Autodesk Fusion 360 part; units mm, degrees
(part 2 of 3)
pattern_linear "Serie R1" count 32 spacing 6 along (-1, 0, 0) count 32 spacing 6 along (0, 1, 0) of bodies 2 makes body 3 at (85.6178, -93.5827, 13.8667) makes body 4 at (79.6178, -93.5827, 13.8667) makes body 5 at (73.6178, -93.5827, 13.8667) makes body 6 at (67.6178, -93.5827, 13.8667) makes body 7 at (61.6178, -93.5827, 13.8667) makes body 8 at (55.6178, -93.5827, 13.8667) makes body 9 at (49.6178, -93.5827, 13.8667) makes body 10 at (43.6178, -93.5827, 13.8667) makes body 11 at (37.6178, -93.5827, 13.8667) makes body 12 at (31.6178, -93.5827, 13.8667) makes body 13 at (25.6178, -93.5827, 13.8667) makes body 14 at (19.6178, -93.5827, 13.8667) makes body 15 at (13.6178, -93.5827, 13.8667) makes body 16 at (10.4095, -93.513, 13.8667) makes body 17 at (4.4095, -93.513, 13.8667) makes body 18 at (-1.5905, -93.513, 13.8667) makes body 19 at (-10.3822, -93.5827, 13.8667) makes body 20 at (-16.3822, -93.5827, 13.8667) makes body 21 at (-22.3822, -93.5827, 13.8667) makes body 22 at (-28.3822, -93.5827, 13.8667) makes body 23 at (-34.3822, -93.5827, 13.8667) makes body 24 at (-40.3822, -93.5827, 13.8667) makes body 25 at (-46.3822, -93.5827, 13.8667) makes body 26 at (-52.3822, -93.5827, 13.8667) makes body 27 at (-58.3822, -93.5827, 13.8667) makes body 28 at (-64.3822, -93.5827, 13.8667) makes body 29 at (-70.3822, -93.5827, 13.8667) makes body 30 at (-76.3822, -93.5827, 13.8667) makes body 31 at (-82.3822, -93.5827, 13.8667) makes body 32 at (-88.3822, -93.5827, 13.8667) makes body 33 at (-94.3822, -93.5827, 13.8667) makes body 34 at (91.6178, -87.5827, 13.8667) makes body 35 at (85.6178, -87.5827, 13.8667) makes body 36 at (79.6178, -87.5827, 13.8667) makes body 37 at (73.6178, -87.5827, 13.8667) makes body 38 at (67.6178, -87.5827, 13.8667) makes body 39 at (61.6178, -87.5827, 13.8667) makes body 40 at (55.6178, -87.5827, 13.8667) makes body 41 at (49.6178, -87.5827, 13.8667) makes body 42 at (43.6178, -87.5827, 13.8667) makes body 43 at (37.6178, -87.5827, 13.8667) makes body 44 at (31.6178, -87.5827, 13.8667) makes body 45 at (25.6178, -87.5827, 13.8667) makes body 46 at (19.6178, -87.5827, 13.8667) makes body 47 at (13.6178, -87.5827, 13.8667) makes body 48 at (10.4095, -87.513, 13.8667) makes body 49 at (4.4095, -87.513, 13.8667) makes body 50 at (-1.5905, -87.513, 13.8667) makes body 51 at (-10.3822, -87.5827, 13.8667) makes body 52 at (-16.3822, -87.5827, 13.8667) makes body 53 at (-22.3822, -87.5827, 13.8667) makes body 54 at (-28.3822, -87.5827, 13.8667) makes body 55 at (-34.3822, -87.5827, 13.8667) makes body 56 at (-40.3822, -87.5827, 13.8667) makes body 57 at (-46.3822, -87.5827, 13.8667) makes body 58 at (-52.3822, -87.5827, 13.8667) makes body 59 at (-58.3822, -87.5827, 13.8667) makes body 60 at (-64.3822, -87.5827, 13.8667) makes body 61 at (-70.3822, -87.5827, 13.8667) makes body 62 at (-76.3822, -87.5827, 13.8667) makes body 63 at (-82.3822, -87.5827, 13.8667) makes body 64 at (-88.3822, -87.5827, 13.8667) makes body 65 at (-94.3822, -87.5827, 13.8667) makes body 66 at (91.6178, -81.5827, 13.8667) makes body 67 at (85.6178, -81.5827, 13.8667) makes body 68 at (79.6178, -81.5827, 13.8667) makes body 69 at (73.6178, -81.5827, 13.8667) makes body 70 at (67.6178, -81.5827, 13.8667) makes body 71 at (61.6178, -81.5827, 13.8667) makes body 72 at (55.6178, -81.5827, 13.8667) makes body 73 at (49.6178, -81.5827, 13.8667) makes body 74 at (43.6178, -81.5827, 13.8667) makes body 75 at (37.6178, -81.5827, 13.8667) makes body 76 at (31.6178, -81.5827, 13.8667) makes body 77 at (25.6178, -81.5827, 13.8667) makes body 78 at (19.6178, -81.5827, 13.8667) makes body 79 at (13.6178, -81.5827, 13.8667) makes body 80 at (10.4095, -81.513, 13.8667) makes body 81 at (4.4095, -81.513, 13.8667) makes body 82 at (-1.5905, -81.513, 13.8667) makes body 83 at (-10.3822, -81.5827, 13.8667) makes body 84 at (-16.3822, -81.5827, 13.8667) makes body 85 at (-22.3822, -81.5827, 13.8667) makes body 86 at (-28.3822, -81.5827, 13.8667) makes body 87 at (-34.3822, -81.5827, 13.8667) makes body 88 at (-40.3822, -81.5827, 13.8667) makes body 89 at (-46.3822, -81.5827, 13.8667) makes body 90 at (-52.3822, -81.5827, 13.8667) makes body 91 at (-58.3822, -81.5827, 13.8667) makes body 92 at (-64.3822, -81.5827, 13.8667) makes body 93 at (-70.3822, -81.5827, 13.8667) makes body 94 at (-76.3822, -81.5827, 13.8667) makes body 95 at (-82.3822, -81.5827, 13.8667) makes body 96 at (-88.3822, -81.5827, 13.8667) makes body 97 at (-94.3822, -81.5827, 13.8667) makes body 98 at (91.6178, -75.5827, 13.8667) makes body 99 at (85.6178, -75.5827, 13.8667) makes body 100 at (79.6178, -75.5827, 13.8667) makes body 101 at (73.6178, -75.5827, 13.8667) makes body 102 at (67.6178, -75.5827, 13.8667) makes body 103 at (61.6178, -75.5827, 13.8667) makes body 104 at (55.6178, -75.5827, 13.8667) makes body 105 at (49.6178, -75.5827, 13.8667) makes body 106 at (43.6178, -75.5827, 13.8667) makes body 107 at (37.6178, -75.5827, 13.8667) makes body 108 at (31.6178, -75.5827, 13.8667) makes body 109 at (25.6178, -75.5827, 13.8667) makes body 110 at (19.6178, -75.5827, 13.8667) makes body 111 at (13.6178, -75.5827, 13.8667) makes body 112 at (10.4095, -75.513, 13.8667) makes body 113 at (4.4095, -75.513, 13.8667) makes body 114 at (-1.5905, -75.513, 13.8667) makes body 115 at (-10.3822, -75.5827, 13.8667) makes body 116 at (-16.3822, -75.5827, 13.8667) makes body 117 at (-22.3822, -75.5827, 13.8667) makes body 118 at (-28.3822, -75.5827, 13.8667) makes body 119 at (-34.3822, -75.5827, 13.8667) makes body 120 at (-40.3822, -75.5827, 13.8667) makes body 121 at (-46.3822, -75.5827, 13.8667) makes body 122 at (-52.3822, -75.5827, 13.8667) makes body 123 at (-58.3822, -75.5827, 13.8667) makes body 124 at (-64.3822, -75.5827, 13.8667) makes body 125 at (-70.3822, -75.5827, 13.8667) makes body 126 at (-76.3822, -75.5827, 13.8667) makes body 127 at (-82.3822, -75.5827, 13.8667) makes body 128 at (-88.3822, -75.5827, 13.8667) makes body 129 at (-94.3822, -75.5827, 13.8667) makes body 130 at (91.6178, -69.5827, 13.8667) makes body 131 at (85.6178, -69.5827, 13.8667) makes body 132 at (79.6178, -69.5827, 13.8667) makes body 133 at (73.6178, -69.5827, 13.8667) makes body 134 at (67.6178, -69.5827, 13.8667) makes body 135 at (61.6178, -69.5827, 13.8667) makes body 136 at (55.6178, -69.5827, 13.8667) makes body 137 at (49.6178, -69.5827, 13.8667) makes body 138 at (43.6178, -69.5827, 13.8667) makes body 139 at (37.6178, -69.5827, 13.8667) makes body 140 at (31.6178, -69.5827, 13.8667) makes body 141 at (25.6178, -69.5827, 13.8667) makes body 142 at (19.6178, -69.5827, 13.8667) makes body 143 at (13.6178, -69.5827, 13.8667) makes body 144 at (10.4095, -69.513, 13.8667) makes body 145 at (4.4095, -69.513, 13.8667) makes body 146 at (-1.5905, -69.513, 13.8667) makes body 147 at (-10.3822, -69.5827, 13.8667) makes body 148 at (-16.3822, -69.5827, 13.8667) makes body 149 at (-22.3822, -69.5827, 13.8667) makes body 150 at (-28.3822, -69.5827, 13.8667) makes body 151 at (-34.3822, -69.5827, 13.8667) makes body 152 at (-40.3822, -69.5827, 13.8667) makes body 153 at (-46.3822, -69.5827, 13.8667) makes body 154 at (-52.3822, -69.5827, 13.8667) makes body 155 at (-58.3822, -69.5827, 13.8667) makes body 156 at (-64.3822, -69.5827, 13.8667) makes body 157 at (-70.3822, -69.5827, 13.8667) makes body 158 at (-76.3822, -69.5827, 13.8667) makes body 159 at (-82.3822, -69.5827, 13.8667) makes body 160 at (-88.3822, -69.5827, 13.8667) makes body 161 at (-94.3822, -69.5827, 13.8667) makes body 162 at (94.3822, -62.4173, 13.8667) makes body 163 at (88.3822, -62.4173, 13.8667) makes body 164 at (82.3822, -62.4173, 13.8667) makes body 165 at (76.3822, -62.4173, 13.8667) makes body 166 at (70.3822, -62.4173, 13.8667) makes body 167 at (64.3822, -62.4173, 13.8667) makes body 168 at (58.3822, -62.4173, 13.8667) makes body 169 at (52.3822, -62.4173, 13.8667) makes body 170 at (46.3822, -62.4173, 13.8667) makes body 171 at (40.3822, -62.4173, 13.8667) makes body 172 at (34.3822, -62.4173, 13.8667) makes body 173 at (28.3822, -62.4173, 13.8667) makes body 174 at (22.3822, -62.4173, 13.8667) makes body 175 at (16.3822, -62.4173, 13.8667) makes body 176 at (10.3822, -62.4173, 13.8667) makes body 177 at (4.3822, -62.4173, 13.8667) makes body 178 at (-1.6178, -62.4173, 13.8667) makes body 179 at (-7.6178, -62.4173, 13.8667) makes body 180 at (-13.6178, -62.4173, 13.8667) makes body 181 at (-19.6178, -62.4173, 13.8667) makes body 182 at (-25.6178, -62.4173, 13.8667) makes body 183 at (-31.6178, -62.4173, 13.8667) makes body 184 at (-37.6178, -62.4173, 13.8667) makes body 185 at (-43.6178, -62.4173, 13.8667) makes body 186 at (-49.6178, -62.4173, 13.8667) makes body 187 at (-55.6178, -62.4173, 13.8667) makes body 188 at (-61.6178, -62.4173, 13.8667) makes body 189 at (-67.6178, -62.4173, 13.8667) makes body 190 at (-73.6178, -62.4173, 13.8667) makes body 191 at (-79.6178, -62.4173, 13.8667) makes body 192 at (-85.6178, -62.4173, 13.8667) makes body 193 at (-91.6178, -62.4173, 13.8667) makes body 194 at (94.3822, -56.4173, 13.8667) makes body 195 at (88.3822, -56.4173, 13.8667) makes body 196 at (82.3822, -56.4173, 13.8667) makes body 197 at (76.3822, -56.4173, 13.8667) makes body 198 at (70.3822, -56.4173, 13.8667) makes body 199 at (64.3822, -56.4173, 13.8667) makes body 200 at (58.3822, -56.4173, 13.8667) makes body 201 at (52.3822, -56.4173, 13.8667) makes body 202 at (46.3822, -56.4173, 13.8667) makes body 203 at (40.3822, -56.4173, 13.8667) makes body 204 at (34.3822, -56.4173, 13.8667) makes body 205 at (28.3822, -56.4173, 13.8667) makes body 206 at (22.3822, -56.4173, 13.8667) makes body 207 at (16.3822, -56.4173, 13.8667) makes body 208 at (10.3822, -56.4173, 13.8667) makes body 209 at (4.3822, -56.4173, 13.8667) makes body 210 at (-1.6178, -56.4173, 13.8667) makes body 211 at (-7.6178, -56.4173, 13.8667) makes body 212 at (-13.6178, -56.4173, 13.8667) makes body 213 at (-19.6178, -56.4173, 13.8667) makes body 214 at (-25.6178, -56.4173, 13.8667) makes body 215 at (-31.6178, -56.4173, 13.8667) makes body 216 at (-37.6178, -56.4173, 13.8667) makes body 217 at (-43.6178, -56.4173, 13.8667) makes body 218 at (-49.6178, -56.4173, 13.8667) makes body 219 at (-55.6178, -56.4173, 13.8667) makes body 220 at (-61.6178, -56.4173, 13.8667) makes body 221 at (-67.6178, -56.4173, 13.8667) makes body 222 at (-73.6178, -56.4173, 13.8667) makes body 223 at (-79.6178, -56.4173, 13.8667) makes body 224 at (-85.6178, -56.4173, 13.8667) makes body 225 at (-91.6178, -56.4173, 13.8667) makes body 226 at (94.3822, -50.4173, 13.8667) makes body 227 at (88.3822, -50.4173, 13.8667) makes body 228 at (82.3822, -50.4173, 13.8667) makes body 229 at (76.3822, -50.4173, 13.8667) makes body 230 at (70.3822, -50.4173, 13.8667) makes body 231 at (64.3822, -50.4173, 13.8667) makes body 232 at (58.3822, -50.4173, 13.8667) makes body 233 at (52.3822, -50.4173, 13.8667) makes body 234 at (46.3822, -50.4173, 13.8667) makes body 235 at (40.3822, -50.4173, 13.8667) makes body 236 at (34.3822, -50.4173, 13.8667) makes body 237 at (28.3822, -50.4173, 13.8667) makes body 238 at (22.3822, -50.4173, 13.8667) makes body 239 at (16.3822, -50.4173, 13.8667) makes body 240 at (10.3822, -50.4173, 13.8667) makes body 241 at (4.3822, -50.4173, 13.8667) makes body 242 at (-1.6178, -50.4173, 13.8667) makes body 243 at (-7.6178, -50.4173, 13.8667) makes body 244 at (-13.6178, -50.4173, 13.8667) makes body 245 at (-19.6178, -50.4173, 13.8667) makes body 246 at (-25.6178, -50.4173, 13.8667) makes body 247 at (-31.6178, -50.4173, 13.8667) makes body 248 at (-37.6178, -50.4173, 13.8667) makes body 249 at (-43.6178, -50.4173, 13.8667) makes body 250 at (-49.6178, -50.4173, 13.8667) makes body 251 at (-55.6178, -50.4173, 13.8667) makes body 252 at (-61.6178, -50.4173, 13.8667) makes body 253 at (-67.6178, -50.4173, 13.8667) makes body 254 at (-73.6178, -50.4173, 13.8667) makes body 255 at (-79.6178, -50.4173, 13.8667) makes body 256 at (-85.6178, -50.4173, 13.8667) makes body 257 at (-91.6178, -50.4173, 13.8667) makes body 258 at (94.3822, -44.4173, 13.8667) makes body 259 at (88.3822, -44.4173, 13.8667) makes body 260 at (82.3822, -44.4173, 13.8667) makes body 261 at (76.3822, -44.4173, 13.8667) makes body 262 at (70.3822, -44.4173, 13.8667) makes body 263 at (64.3822, -44.4173, 13.8667) makes body 264 at (58.3822, -44.4173, 13.8667) makes body 265 at (52.3822, -44.4173, 13.8667) makes body 266 at (46.3822, -44.4173, 13.8667) makes body 267 at (40.3822, -44.4173, 13.8667) makes body 268 at (34.3822, -44.4173, 13.8667) makes body 269 at (28.3822, -44.4173, 13.8667) makes body 270 at (22.3822, -44.4173, 13.8667) makes body 271 at (16.3822, -44.4173, 13.8667) makes body 272 at (10.3822, -44.4173, 13.8667) makes body 273 at (4.3822, -44.4173, 13.8667) makes body 274 at (-1.6178, -44.4173, 13.8667) makes body 275 at (-7.6178, -44.4173, 13.8667) makes body 276 at (-13.6178, -44.4173, 13.8667) makes body 277 at (-19.6178, -44.4173, 13.8667) makes body 278 at (-25.6178, -44.4173, 13.8667) makes body 279 at (-31.6178, -44.4173, 13.8667) makes body 280 at (-37.6178, -44.4173, 13.8667) makes body 281 at (-43.6178, -44.4173, 13.8667) makes body 282 at (-49.6178, -44.4173, 13.8667) makes body 283 at (-55.6178, -44.4173, 13.8667) makes body 284 at (-61.6178, -44.4173, 13.8667) makes body 285 at (-67.6178, -44.4173, 13.8667) makes body 286 at (-73.6178, -44.4173, 13.8667) makes body 287 at (-79.6178, -44.4173, 13.8667) makes body 288 at (-85.6178, -44.4173, 13.8667) makes body 289 at (-91.6178, -44.4173, 13.8667) makes body 290 at (94.3822, -38.4173, 13.8667) makes body 291 at (88.3822, -38.4173, 13.8667) makes body 292 at (82.3822, -38.4173, 13.8667) makes body 293 at (76.3822, -38.4173, 13.8667) makes body 294 at (70.3822, -38.4173, 13.8667) makes body 295 at (64.3822, -38.4173, 13.8667) makes body 296 at (58.3822, -38.4173, 13.8667) makes body 297 at (52.3822, -38.4173, 13.8667) makes body 298 at (46.3822, -38.4173, 13.8667) makes body 299 at (40.3822, -38.4173, 13.8667) makes body 300 at (34.3822, -38.4173, 13.8667) makes body 301 at (28.3822, -38.4173, 13.8667) makes body 302 at (22.3822, -38.4173, 13.8667) makes body 303 at (16.3822, -38.4173, 13.8667) makes body 304 at (10.3822, -38.4173, 13.8667) makes body 305 at (4.3822, -38.4173, 13.8667) makes body 306 at (-1.6178, -38.4173, 13.8667) makes body 307 at (-7.6178, -38.4173, 13.8667) makes body 308 at (-13.6178, -38.4173, 13.8667) makes body 309 at (-19.6178, -38.4173, 13.8667) makes body 310 at (-25.6178, -38.4173, 13.8667) makes body 311 at (-31.6178, -38.4173, 13.8667) makes body 312 at (-37.6178, -38.4173, 13.8667) makes body 313 at (-43.6178, -38.4173, 13.8667) makes body 314 at (-49.6178, -38.4173, 13.8667) makes body 315 at (-55.6178, -38.4173, 13.8667) makes body 316 at (-61.6178, -38.4173, 13.8667) makes body 317 at (-67.6178, -38.4173, 13.8667) makes body 318 at (-73.6178, -38.4173, 13.8667) makes body 319 at (-79.6178, -38.4173, 13.8667) makes body 320 at (-85.6178, -38.4173, 13.8667) makes body 321 at (-91.6178, -38.4173, 13.8667) makes body 322 at (94.3822, -32.4173, 13.8667) makes body 323 at (88.3822, -32.4173, 13.8667) makes body 324 at (82.3822, -32.4173, 13.8667) makes body 325 at (76.3822, -32.4173, 13.8667) makes body 326 at (70.3822, -32.4173, 13.8667) makes body 327 at (64.3822, -32.4173, 13.8667) makes body 328 at (58.3822, -32.4173, 13.8667) makes body 329 at (52.3822, -32.4173, 13.8667) makes body 330 at (46.3822, -32.4173, 13.8667) makes body 331 at (40.3822, -32.4173, 13.8667) makes body 332 at (34.3822, -32.4173, 13.8667) makes body 333 at (28.3822, -32.4173, 13.8667) makes body 334 at (22.3822, -32.4173, 13.8667) makes body 335 at (16.3822, -32.4173, 13.8667) makes body 336 at (10.3822, -32.4173, 13.8667) makes body 337 at (4.3822, -32.4173, 13.8667) makes body 338 at (-1.6178, -32.4173, 13.8667) makes body 339 at (-7.6178, -32.4173, 13.8667) makes body 340 at (-13.6178, -32.4173, 13.8667) makes body 341 at (-19.6178, -32.4173, 13.8667) makes body 342 at (-25.6178, -32.4173, 13.8667) makes body 343 at (-31.6178, -32.4173, 13.8667) makes body 344 at (-37.6178, -32.4173, 13.8667) makes body 345 at (-43.6178, -32.4173, 13.8667) makes body 346 at (-49.6178, -32.4173, 13.8667) makes body 347 at (-55.6178, -32.4173, 13.8667) makes body 348 at (-61.6178, -32.4173, 13.8667) makes body 349 at (-67.6178, -32.4173, 13.8667) makes body 350 at (-73.6178, -32.4173, 13.8667) makes body 351 at (-79.6178, -32.4173, 13.8667) makes body 352 at (-85.6178, -32.4173, 13.8667) makes body 353 at (-91.6178, -32.4173, 13.8667) makes body 354 at (92.0075, -28.1247, 13.8667) makes body 355 at (86.0075, -28.1247, 13.8667) makes body 356 at (80.0075, -28.1247, 13.8667) makes body 357 at (74.0075, -28.1247, 13.8667) makes body 358 at (68.0075, -28.1247, 13.8667) makes body 359 at (62.5937, -28.4439, 13.8667) makes body 360 at (56.5937, -28.4439, 13.8667) makes body 361 at (50.5937, -28.4439, 13.8667) makes body 362 at (44.5937, -28.4439, 13.8667) makes body 363 at (38.5937, -28.4439, 13.8667) makes body 364 at (32.5937, -28.4439, 13.8667) makes body 365 at (28.4925, -26.8506, 13.8667) makes body 366 at (22.4925, -26.8506, 13.8667) makes body 367 at (16.4925, -26.8506, 13.8667) makes body 368 at (10.4925, -26.8506, 13.8667) makes body 369 at (1.5075, -26.8506, 13.5333) makes body 370 at (-4.4925, -26.8506, 13.5333) makes body 371 at (-10.4925, -26.8506, 13.5333) makes body 372 at (-13.5075, -26.8506, 13.8667) makes body 373 at (-19.5075, -26.8506, 13.8667) makes body 374 at (-25.5075, -26.8506, 13.8667) makes body 375 at (-33.4063, -28.4439, 13.8667) makes body 376 at (-39.4063, -28.4439, 13.8667) makes body 377 at (-45.4063, -28.4439, 13.8667) makes body 378 at (-51.4063, -28.4439, 13.8667) makes body 379 at (-57.4063, -28.4439, 13.8667) makes body 380 at (-63.4063, -28.4439, 13.8667) makes body 381 at (-69.9925, -28.1247, 13.8667) makes body 382 at (-75.9925, -28.1247, 13.8667) makes body 383 at (-81.9925, -28.1247, 13.8667) makes body 384 at (-87.9925, -28.1247, 13.8667) makes body 385 at (-93.9925, -28.1247, 13.8667) makes body 386 at (92.0075, -22.1247, 13.8667) makes body 387 at (86.0075, -22.1247, 13.8667) makes body 388 at (80.0075, -22.1247, 13.8667) makes body 389 at (74.0075, -22.1247, 13.8667) makes body 390 at (68.0075, -22.1247, 13.8667) makes body 391 at (62.5937, -22.4439, 13.8667) makes body 392 at (56.5937, -22.4439, 13.8667) makes body 393 at (50.5937, -22.4439, 13.8667) makes body 394 at (44.5937, -22.4439, 13.8667) makes body 395 at (38.5937, -22.4439, 13.8667) makes body 396 at (32.5937, -22.4439, 13.8667) makes body 397 at (28.4925, -20.8506, 13.8667) makes body 398 at (22.4925, -20.8506, 13.8667) makes body 399 at (16.4925, -20.8506, 13.8667) makes body 400 at (10.4925, -20.8506, 13.8667) makes body 401 at (1.5075, -20.8506, 13.5333) makes body 402 at (-4.4925, -20.8506, 13.5333) makes body 403 at (-10.4925, -20.8506, 13.5333) makes body 404 at (-13.5075, -20.8506, 13.8667) makes body 405 at (-19.5075, -20.8506, 13.8667) makes body 406 at (-25.5075, -20.8506, 13.8667) makes body 407 at (-33.4063, -22.4439, 13.8667) makes body 408 at (-39.4063, -22.4439, 13.8667) makes body 409 at (-45.4063, -22.4439, 13.8667) makes body 410 at (-51.4063, -22.4439, 13.8667) makes body 411 at (-57.4063, -22.4439, 13.8667) makes body 412 at (-63.4063, -22.4439, 13.8667) makes body 413 at (-69.9925, -22.1247, 13.8667) makes body 414 at (-75.9925, -22.1247, 13.8667) makes body 415 at (-81.9925, -22.1247, 13.8667) makes body 416 at (-87.9925, -22.1247, 13.8667) makes body 417 at (-93.9925, -22.1247, 13.8667) makes body 418 at (92.0075, -16.1247, 13.8667) makes body 419 at (86.0075, -16.1247, 13.8667) makes body 420 at (80.0075, -16.1247, 13.8667) makes body 421 at (74.0075, -16.1247, 13.8667) makes body 422 at (68.0075, -16.1247, 13.8667) makes body 423 at (62.5937, -16.4439, 13.8667) makes body 424 at (56.5937, -16.4439, 13.8667) makes body 425 at (50.5937, -16.4439, 13.8667) makes body 426 at (44.5937, -16.4439, 13.8667) makes body 427 at (38.5937, -16.4439, 13.8667) makes body 428 at (32.5937, -16.4439, 13.8667) makes body 429 at (25.5075, -14.8506, 13.5333) makes body 430 at (19.5075, -14.8506, 13.5333) makes body 431 at (13.5075, -14.8506, 13.5333) makes body 432 at (7.5075, -14.8506, 13.5333) makes body 433 at (1.5075, -14.8506, 13.5333) makes body 434 at (-4.4925, -14.8506, 13.5333) makes body 435 at (-10.4925, -14.8506, 13.5333) makes body 436 at (-16.4925, -14.8506, 13.5333) makes body 437 at (-22.4925, -14.8506, 13.5333) makes body 438 at (-28.4925, -14.8506, 13.5333) makes body 439 at (-33.4063, -16.4439, 13.8667) makes body 440 at (-39.4063, -16.4439, 13.8667) makes body 441 at (-45.4063, -16.4439, 13.8667) makes body 442 at (-51.4063, -16.4439, 13.8667) makes body 443 at (-57.4063, -16.4439, 13.8667) makes body 444 at (-63.4063, -16.4439, 13.8667) makes body 445 at (-69.9925, -16.1247, 13.8667) makes body 446 at (-75.9925, -16.1247, 13.8667) makes body 447 at (-81.9925, -16.1247, 13.8667) makes body 448 at (-87.9925, -16.1247, 13.8667) makes body 449 at (-93.9925, -16.1247, 13.8667) makes body 450 at (92.5937, -10.4439, 13.8667) makes body 451 at (86.5937, -10.4439, 13.8667) makes body 452 at (80.5937, -10.4439, 13.8667) makes body 453 at (74.5937, -10.4439, 13.8667) makes body 454 at (68.5937, -10.4439, 13.8667) makes body 455 at (62.5937, -10.4439, 13.8667) makes body 456 at (56.5937, -10.4439, 13.8667) makes body 457 at (50.5937, -10.4439, 13.8667) makes body 458 at (44.5937, -10.4439, 13.8667) makes body 459 at (38.5937, -10.4439, 13.8667) makes body 460 at (32.5937, -10.4439, 13.8667) makes body 461 at (25.5075, -8.8506, 13.5333) makes body 462 at (19.5075, -8.8506, 13.5333) makes body 463 at (13.5075, -8.8506, 13.5333) makes body 464 at (7.5075, -8.8506, 13.5333) makes body 465 at (1.5075, -8.8506, 13.5333) makes body 466 at (-4.4925, -8.8506, 13.5333) makes body 467 at (-10.4925, -8.8506, 13.5333) makes body 468 at (-16.4925, -8.8506, 13.5333) makes body 469 at (-22.4925, -8.8506, 13.5333) makes body 470 at (-28.4925, -8.8506, 13.5333) makes body 471 at (-33.4063, -10.4439, 13.8667) makes body 472 at (-39.4063, -10.4439, 13.8667) makes body 473 at (-45.4063, -10.4439, 13.8667) makes body 474 at (-51.4063, -10.4439, 13.8667) makes body 475 at (-57.4063, -10.4439, 13.8667) makes body 476 at (-63.4063, -10.4439, 13.8667) makes body 477 at (-69.4063, -10.4439, 13.8667) makes body 478 at (-75.4063, -10.4439, 13.8667) makes body 479 at (-81.4063, -10.4439, 13.8667) makes body 480 at (-87.4063, -10.4439, 13.8667) makes body 481 at (-93.4063, -10.4439, 13.8667) makes body 482 at (91.5075, -2.8506, 13.5333) makes body 483 at (85.5075, -2.8506, 13.5333) makes body 484 at (79.5075, -2.8506, 13.5333) makes body 485 at (73.5075, -2.8506, 13.5333) makes body 486 at (67.5075, -2.8506, 13.5333) makes body 487 at (62.5937, -4.4439, 13.8667) makes body 488 at (56.5937, -4.4439, 13.8667) makes body 489 at (50.5937, -4.4439, 13.8667) makes body 490 at (44.5937, -4.4439, 13.8667) makes body 491 at (38.5937, -4.4439, 13.8667) makes body 492 at (31.5075, -2.8506, 13.5333) makes body 493 at (25.5075, -2.8506, 13.5333) makes body 494 at (19.5075, -2.8506, 13.5333) makes body 495 at (13.5075, -2.8506, 13.5333) makes body 496 at (7.5075, -2.8506, 13.5333) makes body 497 at (1.5075, -2.8506, 13.5333) makes body 498 at (-4.4925, -2.8506, 13.5333) makes body 499 at (-10.4925, -2.8506, 13.5333) makes body 500 at (-16.4925, -2.8506, 13.5333) makes body 501 at (-22.4925, -2.8506, 13.5333) makes body 502 at (-28.4925, -2.8506, 13.5333) makes body 503 at (-33.4063, -4.4439, 13.8667) makes body 504 at (-39.4063, -4.4439, 13.8667) makes body 505 at (-45.4063, -4.4439, 13.8667) makes body 506 at (-51.4063, -4.4439, 13.8667) makes body 507 at (-57.4063, -4.4439, 13.8667) makes body 508 at (-64.4925, -2.8506, 13.5333) makes body 509 at (-70.4925, -2.8506, 13.5333) makes body 510 at (-76.4925, -2.8506, 13.5333) makes body 511 at (-82.4925, -2.8506, 13.5333) makes body 512 at (-88.4925, -2.8506, 13.5333) makes body 513 at (-94.4925, -2.8506, 13.5333) makes body 514 at (91.5075, 3.1494, 13.5333) makes body 515 at (85.5075, 3.1494, 13.5333) makes body 516 at (79.5075, 3.1494, 13.5333) makes body 517 at (73.5075, 3.1494, 13.5333) makes body 518 at (67.5075, 3.1494, 13.5333) makes body 519 at (62.5937, 1.5561, 13.8667) makes body 520 at (56.5937, 1.5561, 13.8667) makes body 521 at (50.5937, 1.5561, 13.8667) makes body 522 at (44.5937, 1.5561, 13.8667) makes body 523 at (38.5937, 1.5561, 13.8667) makes body 524 at (32.5937, 1.5561, 13.8667) makes body 525 at (25.5075, 3.1494, 13.5333) makes body 526 at (19.5075, 3.1494, 13.5333) makes body 527 at (13.5075, 3.1494, 13.5333) makes body 528 at (7.5075, 3.1494, 13.5333) makes body 529 at (1.5075, 3.1494, 13.5333) makes body 530 at (-4.4925, 3.1494, 13.5333) makes body 531 at (-10.4925, 3.1494, 13.5333) makes body 532 at (-16.4925, 3.1494, 13.5333) makes body 533 at (-22.4925, 3.1494, 13.5333) makes body 534 at (-28.4925, 3.1494, 13.5333) makes body 535 at (-33.4063, 1.5561, 13.8667) makes body 536 at (-39.4063, 1.5561, 13.8667) makes body 537 at (-45.4063, 1.5561, 13.8667) makes body 538 at (-51.4063, 1.5561, 13.8667) makes body 539 at (-57.4063, 1.5561, 13.8667) makes body 540 at (-64.4925, 3.1494, 13.5333) makes body 541 at (-70.4925, 3.1494, 13.5333) makes body 542 at (-76.4925, 3.1494, 13.5333) makes body 543 at (-82.4925, 3.1494, 13.5333) makes body 544 at (-88.4925, 3.1494, 13.5333) makes body 545 at (-94.4925, 3.1494, 13.5333) makes body 546 at (92.5937, 7.5561, 13.8667) makes body 547 at (86.5937, 7.5561, 13.8667) makes body 548 at (80.5937, 7.5561, 13.8667) makes body 549 at (74.5937, 7.5561, 13.8667) makes body 550 at (68.5937, 7.5561, 13.8667) makes body 551 at (62.5937, 7.5561, 13.8667) makes body 552 at (56.5937, 7.5561, 13.8667) makes body 553 at (50.5937, 7.5561, 13.8667) makes body 554 at (44.5937, 7.5561, 13.8667) makes body 555 at (38.5937, 7.5561, 13.8667) makes body 556 at (32.5937, 7.5561, 13.8667) makes body 557 at (25.5075, 9.1494, 13.5333) makes body 558 at (19.5075, 9.1494, 13.5333) makes body 559 at (13.5075, 9.1494, 13.5333) makes body 560 at (7.5075, 9.1494, 13.5333) makes body 561 at (1.5075, 9.1494, 13.5333) makes body 562 at (-4.4925, 9.1494, 13.5333) makes body 563 at (-10.4925, 9.1494, 13.5333) makes body 564 at (-16.4925, 9.1494, 13.5333) makes body 565 at (-22.4925, 9.1494, 13.5333) makes body 566 at (-28.4925, 9.1494, 13.5333) makes body 567 at (-33.4063, 7.5561, 13.8667) makes body 568 at (-39.4063, 7.5561, 13.8667) makes body 569 at (-45.4063, 7.5561, 13.8667) makes body 570 at (-51.4063, 7.5561, 13.8667) makes body 571 at (-57.4063, 7.5561, 13.8667) makes body 572 at (-63.4063, 7.5561, 13.8667) makes body 573 at (-69.4063, 7.5561, 13.8667) makes body 574 at (-75.4063, 7.5561, 13.8667) makes body 575 at (-81.4063, 7.5561, 13.8667) makes body 576 at (-87.4063, 7.5561, 13.8667) makes body 577 at (-93.4063, 7.5561, 13.8667) makes body 578 at (92.5937, 13.5561, 13.8667) makes body 579 at (86.5937, 13.5561, 13.8667) makes body 580 at (80.5937, 13.5561, 13.8667) makes body 581 at (74.5937, 13.5561, 13.8667) makes body 582 at (68.5937, 13.5561, 13.8667) makes body 583 at (61.8043, 15.9057, 13.8667) makes body 584 at (58.1491, 15.9642, 13.8667) makes body 585 at (52.1491, 15.9642, 13.8667) makes body 586 at (46.1491, 15.9642, 13.8667) makes body 587 at (40.1491, 15.9642, 13.8667) makes body 588 at (34.1491, 15.9642, 13.8667) makes body 589 at (25.5075, 15.1494, 13.5333) makes body 590 at (19.5075, 15.1494, 13.5333) makes body 591 at (13.5075, 15.1494, 13.5333) makes body 592 at (7.5075, 15.1494, 13.5333) makes body 593 at (1.5075, 15.1494, 13.5333) makes body 594 at (-4.4925, 15.1494, 13.5333) makes body 595 at (-10.4925, 15.1494, 13.5333) makes body 596 at (-16.4925, 15.1494, 13.5333) makes body 597 at (-22.4925, 15.1494, 13.5333) makes body 598 at (-28.4925, 15.1494, 13.5333) makes body 599 at (-34.1957, 15.9057, 13.8667) makes body 600 at (-37.8509, 15.9642, 13.8667) makes body 601 at (-43.8509, 15.9642, 13.8667) makes body 602 at (-49.8509, 15.9642, 13.8667) makes body 603 at (-55.8509, 15.9642, 13.8667) makes body 604 at (-61.8509, 15.9642, 13.8667) makes body 605 at (-69.4063, 13.5561, 13.8667) makes body 606 at (-75.4063, 13.5561, 13.8667) makes body 607 at (-81.4063, 13.5561, 13.8667) makes body 608 at (-87.4063, 13.5561, 13.8667) makes body 609 at (-93.4063, 13.5561, 13.8667) makes body 610 at (92.0075, 19.8753, 13.8667) makes body 611 at (86.0075, 19.8753, 13.8667) makes body 612 at (80.0075, 19.8753, 13.8667) makes body 613 at (74.0075, 19.8753, 13.8667) makes body 614 at (68.0075, 19.8753, 13.8667) makes body 615 at (62.5937, 19.5561, 13.8667) makes body 616 at (56.5937, 19.5561, 13.8667) makes body 617 at (50.5937, 19.5561, 13.8667) makes body 618 at (44.5937, 19.5561, 13.8667) makes body 619 at (38.5937, 19.5561, 13.8667) makes body 620 at (32.5937, 19.5561, 13.8667) makes body 621 at (28.4925, 21.1494, 13.8667) makes body 622 at (22.4925, 21.1494, 13.8667) makes body 623 at (16.4925, 21.1494, 13.8667) makes body 624 at (10.4925, 21.1494, 13.8667) makes body 625 at (1.5075, 21.1494, 13.5333) makes body 626 at (-4.4925, 21.1494, 13.5333) makes body 627 at (-10.4925, 21.1494, 13.5333) makes body 628 at (-13.5075, 21.1494, 13.8667) makes body 629 at (-19.5075, 21.1494, 13.8667) makes body 630 at (-25.5075, 21.1494, 13.8667) makes body 631 at (-33.4063, 19.5561, 13.8667) makes body 632 at (-39.4063, 19.5561, 13.8667) makes body 633 at (-45.4063, 19.5561, 13.8667) makes body 634 at (-51.4063, 19.5561, 13.8667) makes body 635 at (-57.4063, 19.5561, 13.8667) makes body 636 at (-63.4063, 19.5561, 13.8667) makes body 637 at (-69.9925, 19.8753, 13.8667) makes body 638 at (-75.9925, 19.8753, 13.8667) makes body 639 at (-81.9925, 19.8753, 13.8667) makes body 640 at (-87.9925, 19.8753, 13.8667) makes body 641 at (-93.9925, 19.8753, 13.8667) makes body 642 at (92.0075, 25.8753, 13.8667) makes body 643 at (86.0075, 25.8753, 13.8667) makes body 644 at (80.0075, 25.8753, 13.8667) makes body 645 at (74.0075, 25.8753, 13.8667) makes body 646 at (68.0075, 25.8753, 13.8667) makes body 647 at (62.5937, 25.5561, 13.8667) makes body 648 at (56.5937, 25.5561, 13.8667) makes body 649 at (50.5937, 25.5561, 13.8667) makes body 650 at (44.5937, 25.5561, 13.8667) makes body 651 at (38.5937, 25.5561, 13.8667) makes body 652 at (32.5937, 25.5561, 13.8667) makes body 653 at (28.4925, 27.1494, 13.8667) makes body 654 at (22.4925, 27.1494, 13.8667) makes body 655 at (16.4925, 27.1494, 13.8667) makes body 656 at (10.4925, 27.1494, 13.8667) makes body 657 at (1.5075, 27.1494, 13.5333) makes body 658 at (-4.4925, 27.1494, 13.5333) makes body 659 at (-10.4925, 27.1494, 13.5333) makes body 660 at (-13.5075, 27.1494, 13.8667) makes body 661 at (-19.5075, 27.1494, 13.8667) makes body 662 at (-25.5075, 27.1494, 13.8667) makes body 663 at (-33.4063, 25.5561, 13.8667) makes body 664 at (-39.4063, 25.5561, 13.8667) makes body 665 at (-45.4063, 25.5561, 13.8667) makes body 666 at (-51.4063, 25.5561, 13.8667) makes body 667 at (-57.4063, 25.5561, 13.8667) makes body 668 at (-63.4063, 25.5561, 13.8667) makes body 669 at (-69.9925, 25.8753, 13.8667) makes body 670 at (-75.9925, 25.8753, 13.8667) makes body 671 at (-81.9925, 25.8753, 13.8667) makes body 672 at (-87.9925, 25.8753, 13.8667) makes body 673 at (-93.9925, 25.8753, 13.8667) makes body 674 at (94.3822, 33.5827, 13.8667) makes body 675 at (88.3822, 33.5827, 13.8667) makes body 676 at (82.3822, 33.5827, 13.8667) makes body 677 at (76.3822, 33.5827, 13.8667) makes body 678 at (70.3822, 33.5827, 13.8667) makes body 679 at (64.3822, 33.5827, 13.8667) makes body 680 at (58.3822, 33.5827, 13.8667) makes body 681 at (52.3822, 33.5827, 13.8667) makes body 682 at (46.3822, 33.5827, 13.8667) makes body 683 at (40.3822, 33.5827, 13.8667) makes body 684 at (34.3822, 33.5827, 13.8667) makes body 685 at (28.3822, 33.5827, 13.8667) makes body 686 at (22.3822, 33.5827, 13.8667) makes body 687 at (16.3822, 33.5827, 13.8667) makes body 688 at (10.3822, 33.5827, 13.8667) makes body 689 at (4.3822, 33.5827, 13.8667) makes body 690 at (-1.6178, 33.5827, 13.8667) makes body 691 at (-7.6178, 33.5827, 13.8667) makes body 692 at (-13.6178, 33.5827, 13.8667) makes body 693 at (-19.6178, 33.5827, 13.8667) makes body 694 at (-25.6178, 33.5827, 13.8667) makes body 695 at (-31.6178, 33.5827, 13.8667) makes body 696 at (-37.6178, 33.5827, 13.8667) makes body 697 at (-43.6178, 33.5827, 13.8667) makes body 698 at (-49.6178, 33.5827, 13.8667) makes body 699 at (-55.6178, 33.5827, 13.8667) makes body 700 at (-61.6178, 33.5827, 13.8667) makes body 701 at (-67.6178, 33.5827, 13.8667) makes body 702 at (-73.6178, 33.5827, 13.8667) makes body 703 at (-79.6178, 33.5827, 13.8667) makes body 704 at (-85.6178, 33.5827, 13.8667) makes body 705 at (-91.6178, 33.5827, 13.8667) makes body 706 at (94.3822, 39.5827, 13.8667) makes body 707 at (88.3822, 39.5827, 13.8667) makes body 708 at (82.3822, 39.5827, 13.8667) makes body 709 at (76.3822, 39.5827, 13.8667) makes body 710 at (70.3822, 39.5827, 13.8667) makes body 711 at (64.3822, 39.5827, 13.8667) makes body 712 at (58.3822, 39.5827, 13.8667) makes body 713 at (52.3822, 39.5827, 13.8667) makes body 714 at (46.3822, 39.5827, 13.8667) makes body 715 at (40.3822, 39.5827, 13.8667) makes body 716 at (34.3822, 39.5827, 13.8667) makes body 717 at (28.3822, 39.5827, 13.8667) makes body 718 at (22.3822, 39.5827, 13.8667) makes body 719 at (16.3822, 39.5827, 13.8667) makes body 720 at (10.3822, 39.5827, 13.8667) makes body 721 at (4.3822, 39.5827, 13.8667) makes body 722 at (-1.6178, 39.5827, 13.8667) makes body 723 at (-7.6178, 39.5827, 13.8667) makes body 724 at (-13.6178, 39.5827, 13.8667) makes body 725 at (-19.6178, 39.5827, 13.8667) makes body 726 at (-25.6178, 39.5827, 13.8667) makes body 727 at (-31.6178, 39.5827, 13.8667) makes body 728 at (-37.6178, 39.5827, 13.8667) makes body 729 at (-43.6178, 39.5827, 13.8667) makes body 730 at (-49.6178, 39.5827, 13.8667) makes body 731 at (-55.6178, 39.5827, 13.8667) makes body 732 at (-61.6178, 39.5827, 13.8667) makes body 733 at (-67.6178, 39.5827, 13.8667) makes body 734 at (-73.6178, 39.5827, 13.8667) makes body 735 at (-79.6178, 39.5827, 13.8667) makes body 736 at (-85.6178, 39.5827, 13.8667) makes body 737 at (-91.6178, 39.5827, 13.8667) makes body 738 at (94.3822, 45.5827, 13.8667) makes body 739 at (88.3822, 45.5827, 13.8667) makes body 740 at (82.3822, 45.5827, 13.8667) makes body 741 at (76.3822, 45.5827, 13.8667) makes body 742 at (70.3822, 45.5827, 13.8667) makes body 743 at (64.3822, 45.5827, 13.8667) makes body 744 at (58.3822, 45.5827, 13.8667) makes body 745 at (52.3822, 45.5827, 13.8667) makes body 746 at (46.3822, 45.5827, 13.8667) makes body 747 at (40.3822, 45.5827, 13.8667) makes body 748 at (34.3822, 45.5827, 13.8667) makes body 749 at (28.3822, 45.5827, 13.8667) makes body 750 at (22.3822, 45.5827, 13.8667) makes body 751 at (16.3822, 45.5827, 13.8667) makes body 752 at (10.3822, 45.5827, 13.8667) makes body 753 at (4.3822, 45.5827, 13.8667) makes body 754 at (-1.6178, 45.5827, 13.8667) makes body 755 at (-7.6178, 45.5827, 13.8667) makes body 756 at (-13.6178, 45.5827, 13.8667) makes body 757 at (-19.6178, 45.5827, 13.8667) makes body 758 at (-25.6178, 45.5827, 13.8667) makes body 759 at (-31.6178, 45.5827, 13.8667) makes body 760 at (-37.6178, 45.5827, 13.8667) makes body 761 at (-43.6178, 45.5827, 13.8667) makes body 762 at (-49.6178, 45.5827, 13.8667) makes body 763 at (-55.6178, 45.5827, 13.8667) makes body 764 at (-61.6178, 45.5827, 13.8667) makes body 765 at (-67.6178, 45.5827, 13.8667) makes body 766 at (-73.6178, 45.5827, 13.8667) makes body 767 at (-79.6178, 45.5827, 13.8667) makes body 768 at (-85.6178, 45.5827, 13.8667) makes body 769 at (-91.6178, 45.5827, 13.8667) makes body 770 at (94.3822, 51.5827, 13.8667) makes body 771 at (88.3822, 51.5827, 13.8667) makes body 772 at (82.3822, 51.5827, 13.8667) makes body 773 at (76.3822, 51.5827, 13.8667) makes body 774 at (70.3822, 51.5827, 13.8667) makes body 775 at (64.3822, 51.5827, 13.8667) makes body 776 at (58.3822, 51.5827, 13.8667) makes body 777 at (52.3822, 51.5827, 13.8667) makes body 778 at (46.3822, 51.5827, 13.8667) makes body 779 at (40.3822, 51.5827, 13.8667) makes body 780 at (34.3822, 51.5827, 13.8667) makes body 781 at (28.3822, 51.5827, 13.8667) makes body 782 at (22.3822, 51.5827, 13.8667) makes body 783 at (16.3822, 51.5827, 13.8667) makes body 784 at (10.3822, 51.5827, 13.8667) makes body 785 at (4.3822, 51.5827, 13.8667) makes body 786 at (-1.6178, 51.5827, 13.8667) makes body 787 at (-7.6178, 51.5827, 13.8667) makes body 788 at (-13.6178, 51.5827, 13.8667) makes body 789 at (-19.6178, 51.5827, 13.8667) makes body 790 at (-25.6178, 51.5827, 13.8667) makes body 791 at (-31.6178, 51.5827, 13.8667) makes body 792 at (-37.6178, 51.5827, 13.8667) makes body 793 at (-43.6178, 51.5827, 13.8667) makes body 794 at (-49.6178, 51.5827, 13.8667) makes body 795 at (-55.6178, 51.5827, 13.8667) makes body 796 at (-61.6178, 51.5827, 13.8667) makes body 797 at (-67.6178, 51.5827, 13.8667) makes body 798 at (-73.6178, 51.5827, 13.8667) makes body 799 at (-79.6178, 51.5827, 13.8667) makes body 800 at (-85.6178, 51.5827, 13.8667) makes body 801 at (-91.6178, 51.5827, 13.8667) makes body 802 at (94.3822, 57.5827, 13.8667) makes body 803 at (88.3822, 57.5827, 13.8667) makes body 804 at (82.3822, 57.5827, 13.8667) makes body 805 at (76.3822, 57.5827, 13.8667) makes body 806 at (70.3822, 57.5827, 13.8667) makes body 807 at (64.3822, 57.5827, 13.8667) makes body 808 at (58.3822, 57.5827, 13.8667) makes body 809 at (52.3822, 57.5827, 13.8667) makes body 810 at (46.3822, 57.5827, 13.8667) makes body 811 at (40.3822, 57.5827, 13.8667) makes body 812 at (34.3822, 57.5827, 13.8667) makes body 813 at (28.3822, 57.5827, 13.8667) makes body 814 at (22.3822, 57.5827, 13.8667) makes body 815 at (16.3822, 57.5827, 13.8667) makes body 816 at (10.3822, 57.5827, 13.8667) makes body 817 at (4.3822, 57.5827, 13.8667) makes body 818 at (-1.6178, 57.5827, 13.8667) makes body 819 at (-7.6178, 57.5827, 13.8667) makes body 820 at (-13.6178, 57.5827, 13.8667) makes body 821 at (-19.6178, 57.5827, 13.8667) makes body 822 at (-25.6178, 57.5827, 13.8667) makes body 823 at (-31.6178, 57.5827, 13.8667) makes body 824 at (-37.6178, 57.5827, 13.8667) makes body 825 at (-43.6178, 57.5827, 13.8667) makes body 826 at (-49.6178, 57.5827, 13.8667) makes body 827 at (-55.6178, 57.5827, 13.8667) makes body 828 at (-61.6178, 57.5827, 13.8667) makes body 829 at (-67.6178, 57.5827, 13.8667) makes body 830 at (-73.6178, 57.5827, 13.8667) makes body 831 at (-79.6178, 57.5827, 13.8667) makes body 832 at (-85.6178, 57.5827, 13.8667) makes body 833 at (-91.6178, 57.5827, 13.8667) makes body 834 at (94.3822, 63.5827, 13.8667) makes body 835 at (88.3822, 63.5827, 13.8667) makes body 836 at (82.3822, 63.5827, 13.8667) makes body 837 at (76.3822, 63.5827, 13.8667) makes body 838 at (70.3822, 63.5827, 13.8667) makes body 839 at (64.3822, 63.5827, 13.8667) makes body 840 at (58.3822, 63.5827, 13.8667) makes body 841 at (52.3822, 63.5827, 13.8667) makes body 842 at (46.3822, 63.5827, 13.8667) makes body 843 at (40.3822, 63.5827, 13.8667) makes body 844 at (34.3822, 63.5827, 13.8667) makes body 845 at (28.3822, 63.5827, 13.8667) makes body 846 at (22.3822, 63.5827, 13.8667) makes body 847 at (16.3822, 63.5827, 13.8667) makes body 848 at (10.3822, 63.5827, 13.8667) makes body 849 at (4.3822, 63.5827, 13.8667) makes body 850 at (-1.6178, 63.5827, 13.8667) makes body 851 at (-7.6178, 63.5827, 13.8667) makes body 852 at (-13.6178, 63.5827, 13.8667) makes body 853 at (-19.6178, 63.5827, 13.8667) makes body 854 at (-25.6178, 63.5827, 13.8667) makes body 855 at (-31.6178, 63.5827, 13.8667) makes body 856 at (-37.6178, 63.5827, 13.8667) makes body 857 at (-43.6178, 63.5827, 13.8667) makes body 858 at (-49.6178, 63.5827, 13.8667) makes body 859 at (-55.6178, 63.5827, 13.8667) makes body 860 at (-61.6178, 63.5827, 13.8667) makes body 861 at (-67.6178, 63.5827, 13.8667) makes body 862 at (-73.6178, 63.5827, 13.8667) makes body 863 at (-79.6178, 63.5827, 13.8667) makes body 864 at (-85.6178, 63.5827, 13.8667) makes body 865 at (-91.6178, 63.5827, 13.8667) makes body 866 at (91.6178, 68.4173, 13.8667) makes body 867 at (85.6178, 68.4173, 13.8667) makes body 868 at (79.6178, 68.4173, 13.8667) makes body 869 at (73.6178, 68.4173, 13.8667) makes body 870 at (67.6178, 68.4173, 13.8667) makes body 871 at (61.6178, 68.4173, 13.8667) makes body 872 at (55.6178, 68.4173, 13.8667) makes body 873 at (49.6178, 68.4173, 13.8667) makes body 874 at (43.6178, 68.4173, 13.8667) makes body 875 at (37.6178, 68.4173, 13.8667) makes body 876 at (31.6178, 68.4173, 13.8667) makes body 877 at (25.6178, 68.4173, 13.8667) makes body 878 at (19.6178, 68.4173, 13.8667) makes body 879 at (13.6178, 68.4173, 13.8667) makes body 880 at (10.4095, 68.487, 13.8667) makes body 881 at (4.4095, 68.487, 13.8667) makes body 882 at (-1.5905, 68.487, 13.8667) makes body 883 at (-10.3822, 68.4173, 13.8667) makes body 884 at (-16.3822, 68.4173, 13.8667) makes body 885 at (-22.3822, 68.4173, 13.8667) makes body 886 at (-28.3822, 68.4173, 13.8667) makes body 887 at (-34.3822, 68.4173, 13.8667) makes body 888 at (-40.3822, 68.4173, 13.8667) makes body 889 at (-46.3822, 68.4173, 13.8667) makes body 890 at (-52.3822, 68.4173, 13.8667) makes body 891 at (-58.3822, 68.4173, 13.8667) makes body 892 at (-64.3822, 68.4173, 13.8667) makes body 893 at (-70.3822, 68.4173, 13.8667) makes body 894 at (-76.3822, 68.4173, 13.8667) makes body 895 at (-82.3822, 68.4173, 13.8667) makes body 896 at (-88.3822, 68.4173, 13.8667) makes body 897 at (-94.3822, 68.4173, 13.8667) makes body 898 at (91.6178, 74.4173, 13.8667) makes body 899 at (85.6178, 74.4173, 13.8667) makes body 900 at (79.6178, 74.4173, 13.8667) makes body 901 at (73.6178, 74.4173, 13.8667) makes body 902 at (67.6178, 74.4173, 13.8667) makes body 903 at (61.6178, 74.4173, 13.8667) makes body 904 at (55.6178, 74.4173, 13.8667) makes body 905 at (49.6178, 74.4173, 13.8667) makes body 906 at (43.6178, 74.4173, 13.8667) makes body 907 at (37.6178, 74.4173, 13.8667) makes body 908 at (31.6178, 74.4173, 13.8667) makes body 909 at (25.6178, 74.4173, 13.8667) makes body 910 at (19.6178, 74.4173, 13.8667) makes body 911 at (13.6178, 74.4173, 13.8667) makes body 912 at (10.4095, 74.487, 13.8667) makes body 913 at (4.4095, 74.487, 13.8667) makes body 914 at (-1.5905, 74.487, 13.8667) makes body 915 at (-10.3822, 74.4173, 13.8667) makes body 916 at (-16.3822, 74.4173, 13.8667) makes body 917 at (-22.3822, 74.4173, 13.8667) makes body 918 at (-28.3822, 74.4173, 13.8667) makes body 919 at (-34.3822, 74.4173, 13.8667) makes body 920 at (-40.3822, 74.4173, 13.8667) makes body 921 at (-46.3822, 74.4173, 13.8667) makes body 922 at (-52.3822, 74.4173, 13.8667) makes body 923 at (-58.3822, 74.4173, 13.8667) makes body 924 at (-64.3822, 74.4173, 13.8667) makes body 925 at (-70.3822, 74.4173, 13.8667) makes body 926 at (-76.3822, 74.4173, 13.8667) makes body 927 at (-82.3822, 74.4173, 13.8667) makes body 928 at (-88.3822, 74.4173, 13.8667) makes body 929 at (-94.3822, 74.4173, 13.8667) makes body 930 at (91.6178, 80.4173, 13.8667) makes body 931 at (85.6178, 80.4173, 13.8667) makes body 932 at (79.6178, 80.4173, 13.8667) makes body 933 at (73.6178, 80.4173, 13.8667) makes body 934 at (67.6178, 80.4173, 13.8667) makes body 935 at (61.6178, 80.4173, 13.8667) makes body 936 at (55.6178, 80.4173, 13.8667) makes body 937 at (49.6178, 80.4173, 13.8667) makes body 938 at (43.6178, 80.4173, 13.8667) makes body 939 at (37.6178, 80.4173, 13.8667) makes body 940 at (31.6178, 80.4173, 13.8667) makes body 941 at (25.6178, 80.4173, 13.8667) makes body 942 at (19.6178, 80.4173, 13.8667) makes body 943 at (13.6178, 80.4173, 13.8667) makes body 944 at (10.4095, 80.487, 13.8667) makes body 945 at (4.4095, 80.487, 13.8667) makes body 946 at (-1.5905, 80.487, 13.8667) makes body 947 at (-10.3822, 80.4173, 13.8667) makes body 948 at (-16.3822, 80.4173, 13.8667) makes body 949 at (-22.3822, 80.4173, 13.8667) makes body 950 at (-28.3822, 80.4173, 13.8667) makes body 951 at (-34.3822, 80.4173, 13.8667) makes body 952 at (-40.3822, 80.4173, 13.8667) makes body 953 at (-46.3822, 80.4173, 13.8667) makes body 954 at (-52.3822, 80.4173, 13.8667) makes body 955 at (-58.3822, 80.4173, 13.8667) makes body 956 at (-64.3822, 80.4173, 13.8667) makes body 957 at (-70.3822, 80.4173, 13.8667) makes body 958 at (-76.3822, 80.4173, 13.8667) makes body 959 at (-82.3822, 80.4173, 13.8667) makes body 960 at (-88.3822, 80.4173, 13.8667) makes body 961 at (-94.3822, 80.4173, 13.8667) makes body 962 at (91.6178, 86.4173, 13.8667) makes body 963 at (85.6178, 86.4173, 13.8667) makes body 964 at (79.6178, 86.4173, 13.8667) makes body 965 at (73.6178, 86.4173, 13.8667) makes body 966 at (67.6178, 86.4173, 13.8667) makes body 967 at (61.6178, 86.4173, 13.8667) makes body 968 at (55.6178, 86.4173, 13.8667) makes body 969 at (49.6178, 86.4173, 13.8667) makes body 970 at (43.6178, 86.4173, 13.8667) makes body 971 at (37.6178, 86.4173, 13.8667) makes body 972 at (31.6178, 86.4173, 13.8667) makes body 973 at (25.6178, 86.4173, 13.8667) makes body 974 at (19.6178, 86.4173, 13.8667) makes body 975 at (13.6178, 86.4173, 13.8667) makes body 976 at (10.4095, 86.487, 13.8667) makes body 977 at (4.4095, 86.487, 13.8667) makes body 978 at (-1.5905, 86.487, 13.8667) makes body 979 at (-10.3822, 86.4173, 13.8667) makes body 980 at (-16.3822, 86.4173, 13.8667) makes body 981 at (-22.3822, 86.4173, 13.8667) makes body 982 at (-28.3822, 86.4173, 13.8667) makes body 983 at (-34.3822, 86.4173, 13.8667) makes body 984 at (-40.3822, 86.4173, 13.8667) makes body 985 at (-46.3822, 86.4173, 13.8667) makes body 986 at (-52.3822, 86.4173, 13.8667) makes body 987 at (-58.3822, 86.4173, 13.8667) makes body 988 at (-64.3822, 86.4173, 13.8667) makes body 989 at (-70.3822, 86.4173, 13.8667) makes body 990 at (-76.3822, 86.4173, 13.8667) makes body 991 at (-82.3822, 86.4173, 13.8667) makes body 992 at (-88.3822, 86.4173, 13.8667) makes body 993 at (-94.3822, 86.4173, 13.8667) makes body 994 at (91.6178, 92.4173, 13.8667) makes body 995 at (85.6178, 92.4173, 13.8667) makes body 996 at (79.6178, 92.4173, 13.8667) makes body 997 at (73.6178, 92.4173, 13.8667) makes body 998 at (67.6178, 92.4173, 13.8667) makes body 999 at (61.6178, 92.4173, 13.8667) makes body 1000 at (55.6178, 92.4173, 13.8667) makes body 1001 at (49.6178, 92.4173, 13.8667) makes body 1002 at (43.6178, 92.4173, 13.8667) makes body 1003 at (37.6178, 92.4173, 13.8667) makes body 1004 at (31.6178, 92.4173, 13.8667) makes body 1005 at (25.6178, 92.4173, 13.8667) makes body 1006 at (19.6178, 92.4173, 13.8667) makes body 1007 at (13.6178, 92.4173, 13.8667) makes body 1008 at (10.4095, 92.487, 13.8667) makes body 1009 at (4.4095, 92.487, 13.8667) makes body 1010 at (-1.5905, 92.487, 13.8667) makes body 1011 at (-10.3822, 92.4173, 13.8667) makes body 1012 at (-16.3822, 92.4173, 13.8667) makes body 1013 at (-22.3822, 92.4173, 13.8667) makes body 1014 at (-28.3822, 92.4173, 13.8667) makes body 1015 at (-34.3822, 92.4173, 13.8667) makes body 1016 at (-40.3822, 92.4173, 13.8667) makes body 1017 at (-46.3822, 92.4173, 13.8667) makes body 1018 at (-52.3822, 92.4173, 13.8667) makes body 1019 at (-58.3822, 92.4173, 13.8667) makes body 1020 at (-64.3822, 92.4173, 13.8667) makes body 1021 at (-70.3822, 92.4173, 13.8667) makes body 1022 at (-76.3822, 92.4173, 13.8667) makes body 1023 at (-82.3822, 92.4173, 13.8667) makes body 1024 at (-88.3822, 92.4173, 13.8667) makes body 1025 at (-94.3822, 92.4173, 13.8667)
equation "d21 = ( -6 * 31 ) * 1 mm"
equation "d22 = ( -6 * 31 ) * 1 mm"

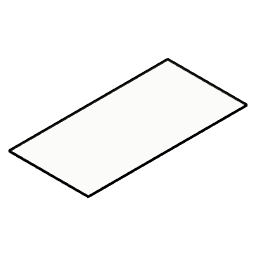
design "vetro"
Autodesk Fusion 360 part; units mm, degrees
sketch "Schizzo1" plane through (0, 0, 0) normal (0, 0, 1) x (1, 0, 0)
  line L0 (-125, 0) -> (125, 0)
  line L1 (125, 0) -> (125, -500)
  line L2 (125, -500) -> (-125, -500)
  line L3 (-125, -500) -> (-125, 0)
  line L4 (0, 0) -> (0, -500) construction
  dimension "d1" = 250
  dimension "d2" = 500
  constraint horizontal L0
  constraint vertical L1
  constraint horizontal L2
  constraint vertical L3
  constraint midpoint L0 L4.start
  constraint midpoint L2 L4.end
  constraint coincident L4.start origin
  measures "d1" distance of L0.start L0.end
  measures "d2" distance of L0.start L2.end
extrude "Estrusione1" add sketch "Schizzo1" along normal blind 4

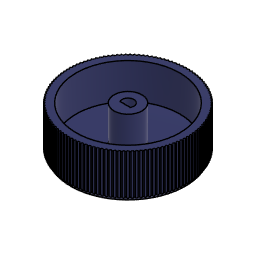
design "pomello"
Autodesk Fusion 360 part; units mm, degrees
sketch "Schizzo1" plane through (0, 0, 0) normal (0, 0, 1) x (1, 0, 0)
  circle A0 centre (0, 0) radius 29
  dimension "d1" = 58
  constraint coincident A0.centre origin
  measures "d1" diameter of A0
extrude "Estrusione1" add sketch "Schizzo1" along normal blind 2 draft 30
extrude "Estrusione2" add 1 faces at (-3.5403, 2.1964, 2) along direction (0, 0, 1) blind 20
sketch "Schizzo2" plane through (0, 0, 22) normal (0, 0, 1) x (-1, 0, 0)
  circle A0 centre (0, 0) radius 30.1547
  circle A1 centre (0, 0) radius 3
  line L0 (11, -3) -> (-17, -3)
  line L1 (-17, -3) -> (-17, 1.4)
  line L2 (-17, 1.4) -> (11, 1.4)
  line L3 (11, 1.4) -> (11, -3)
  dimension "d6" = 6
  dimension "d7" = 4.4
  constraint coincident A0.centre A1.centre
  constraint horizontal L0
  constraint vertical L1
  constraint horizontal L2
  constraint vertical L3
  constraint tangent A1 L0
  measures "d6" diameter of A1
  measures "d7" distance of L0.start L2.end
extrude "Estrusione3" cut sketch "Schizzo2" against normal blind 12 contours A1 L2 picked at (-0.8946, -0.4352)